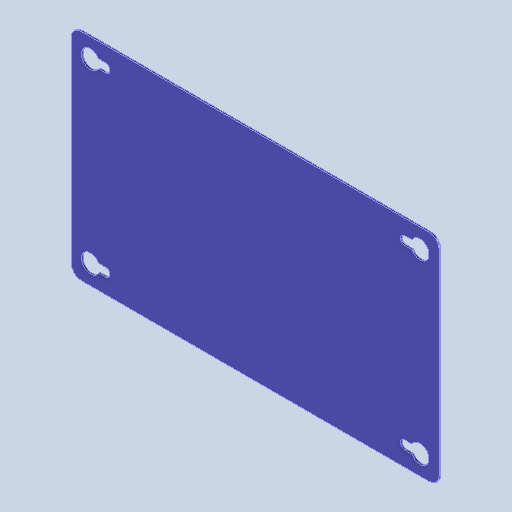
# Autodesk Inventor part: TorsoBackColorMarker
Saved by Autodesk Inventor 2024.2 (Build 282272000, 272)
## iProperties
Created: 2024-01-22
Part Number: TorsoBackColorMarker
Material: Polypropylene
Document SubType Name: Modeling
Designer: Masato Kubotera
Density: 0.899 g/cm^3
Appearance: Smooth - Navy
Mass: 16.5888 g
Surface Area: 500.852 cm^2
Volume: 18.4525 cm^3
Author: Masato Kubotera
Autodesk Inventor part; units mm, degrees
ref_plane "YZ Plane" through (0, 0, 0) normal (1, 0, 0) x (0, 1, 0)
ref_plane "XZ Plane" through (0, 0, 0) normal (0, 1, 0) x (-1, 0, 0)
ref_plane "XY Plane" through (0, 0, 0) normal (0, 0, 1) x (1, 0, 0)
derived "TorsoElectronicBoxBackFrame.ipt"
sketch "Sketch8" plane through (0, 0, 0) normal (1, 0, 0) x (0, 1, 0)
  arc A0 (76.5201, -23.6) -> (76.5201, -19.4) centre (80.5, -21.5) ccw projected
  line L0 (73, -19.4) -> (76.5201, -19.4) projected
  arc A1 (73, -19.4) -> (73, -23.6) centre (73, -21.5) ccw projected
  line L1 (73, -23.6) -> (76.5201, -23.6) projected
  line L2 (90, 74.5) -> (90, -74.5) projected
  line L3 (90, -31) -> (-90, -31) projected
  line L4 (-90, 74.5) -> (90, 74.5) projected
  line L5 (73, 67.1) -> (76.5201, 67.1) projected
  arc A2 (73, 67.1) -> (73, 62.9) centre (73, 65) ccw projected
  arc A3 (76.5201, 62.9) -> (76.5201, 67.1) centre (80.5, 65) ccw projected
  line L6 (73, 62.9) -> (76.5201, 62.9) projected
  line L7 (0, 74.5) -> (0, -74.5) projected
  arc A4 (-76.5201, -19.4) -> (-76.5201, -23.6) centre (-80.5, -21.5) ccw
  line L8 (-73, -19.4) -> (-76.5201, -19.4)
  arc A5 (-73, -23.6) -> (-73, -19.4) centre (-73, -21.5) ccw
  line L9 (-73, -23.6) -> (-76.5201, -23.6)
  line L10 (-73, 67.1) -> (-76.5201, 67.1)
  arc A6 (-73, 62.9) -> (-73, 67.1) centre (-73, 65) ccw
  arc A7 (-76.5201, 67.1) -> (-76.5201, 62.9) centre (-80.5, 65) ccw
  line L11 (-73, 62.9) -> (-76.5201, 62.9)
  line L12 (-90, -74.5) -> (-90, 74.5) projected
  point P0 (0, 0)
  constraints: 14 symmetric about line, 8 end point, 8 point on circle, 4 centre point, 4 other
extrude "Extrusion1" add sketch "Sketch8" along normal blind 0.75
fillet "R5" radius 5 4 edges at (0.375, -90, 74.5) (0.375, -90, -31) (0.375, 90, 74.5) (0.375, 90, -31)
sketch "Sketch1" plane through (0, 0, 0) normal (1, 0, 0) x (0, 1, 0)
  line L0 (-90, 74.5) -> (90, 74.5) projected
  line L1 (90, 74.5) -> (90, -74.5) projected
  line L2 (90, -74.5) -> (-90, -74.5) projected
  line L3 (-90, -74.5) -> (-90, 74.5) projected
  line L4 (-90, 74.5) -> (90, -74.5) construction
  line L5 (90, 74.5) -> (-90, -74.5) construction
  line L6 (85, 74.5) -> (85, 46.75) projected
  line L7 (85, 46.75) -> (90, 46.75) projected
  line L8 (0, 74.5) -> (0, -74.5) projected
  line L9 (90, 0) -> (-90, 0) construction
  arc A0 (85, 49.75) -> (85, 46.75) centre (85, 48.25) ccw projected
  line L10 (-90, 74.5) -> (-90, -74.5) projected
  circle A1 centre (73, 65) radius 3 construction
  arc A2 (73, 67.1) -> (73, 62.9) centre (73, 65) ccw construction
  line L11 (73, 67.1) -> (76.5201, 67.1) construction
  arc A3 (76.5201, 62.9) -> (76.5201, 67.1) centre (80.5, 65) ccw construction
  line L12 (73, 65) -> (80.5, 65) construction
  line L13 (73, 62.9) -> (76.5201, 62.9) construction
  line L14 (90, 28.75) -> (85, 28.75) construction
  line L15 (90, 14.75) -> (85, 14.75) construction
  line L16 (90, 21.75) -> (85, 21.75) construction
  line L17 (85, -3.25) -> (90, -3.25) projected
  arc A4 (85, -3.25) -> (85, -6.25) centre (85, -4.75) ccw projected
  line L18 (85, -6.25) -> (85, -74.5) projected
  line L19 (90, -31) -> (-90, -31) projected
  line L20 (74, -31) -> (74, -74.5) projected
  line L21 (-90, 21.75) -> (90, 21.75) construction
  circle A5 centre (73, -21.5) radius 3 construction
  arc A6 (73, -19.4) -> (73, -23.6) centre (73, -21.5) ccw construction
  line L22 (73, -23.6) -> (76.5201, -23.6) construction
  arc A7 (76.5201, -23.6) -> (76.5201, -19.4) centre (80.5, -21.5) ccw construction
  line L23 (73, -21.5) -> (80.5, -21.5) construction
  line L24 (73, -19.4) -> (76.5201, -19.4) construction
  arc A8 (74, -31) -> (74, -34) centre (74, -32.5) ccw projected
  point P0 (0, 0)
  point P1 (85, -74.5)
  point P2 (85, 65)
  point P3 (85, -21.5)
  constraints: 1 other
body "Solid2"
